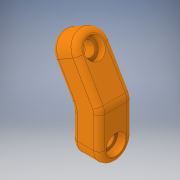
# Autodesk Inventor part: Link2
Saved by Autodesk Inventor 2019 (Build 230136000, 136)
## iProperties
Created: 2022-07-14
Part Number: Link2
Material: Generic
Document SubType Name: Modeling
Designer: zreik
Density: 1 g/cm^3
Appearance: Orange
d46: 10.000 mm
Author: zreik
Autodesk Inventor part; units mm, degrees
ref_plane "YZ Plane" through (0, 0, 0) normal (1, 0, 0) x (0, 1, 0)
ref_plane "XZ Plane" through (0, 0, 0) normal (0, 1, 0) x (-1, 0, 0)
ref_plane "XY Plane" through (0, 0, 0) normal (0, 0, 1) x (1, 0, 0)
sketch "Sketch1" plane through (0, 0, 0) normal (0, 0, 1) x (1, 0, 0)
  line L0 (53.3205, 0) -> (0, 0)
  line L1 (0, 0) -> (60.3287, 34.8308)
  line L2 (43.3205, 0) -> (43.3205, 8.6603)
  line L3 (42.6506, 11.1603) -> (36.8205, 21.2583)
  line L4 (53.3205, 0) -> (53.3205, 11.3397)
  line L5 (52.6506, 13.8397) -> (45.4808, 26.2583)
  arc A0 (43.3205, 8.6603) -> (42.6506, 11.1603) centre (38.3205, 8.6603) ccw
  arc A1 (53.3205, 11.3397) -> (52.6506, 13.8397) centre (48.3205, 11.3397) ccw
  line L6 (45.4808, 26.2583) -> (36.8205, 21.2583)
  line L7 (45.4808, 26.2583) -> (52.6506, 13.8397)
  line L8 (36.8205, 21.2583) -> (42.6506, 11.1603)
  line L9 (43.3205, 0) -> (53.3205, 0)
  line L10 (53.3205, 0) -> (53.3205, 11.3397)
  line L11 (43.3205, 0) -> (53.3205, 0)
  line L12 (53.3205, 0) -> (53.3205, 11.3397)
  line L13 (52.6506, 13.8397) -> (45.4808, 26.2583)
  line L14 (45.4808, 26.2583) -> (36.8205, 21.2583)
  line L15 (36.8205, 21.2583) -> (42.6506, 11.1603)
  line L16 (43.3205, 8.6603) -> (43.3205, 0)
  point P0 (43.3013, 25)
  point P1 (43.3205, 10)
  dimension "d37" = 30
  dimension "d38" = 10
  dimension "d39" = 10
  dimension "d40" = 0
  dimension "d41" = 0
  dimension "d42" = 10
  dimension "d43" = 13
  dimension "d44" = 150
  dimension "d45" = 5
  constraints: 34 end point, 9 collinear, 6 point on line, 4 point on circle, 4 tangent, 2 centre point, 2 parallel, 1 coincident, 1 equal radius, 1 horizontal, 1 vertical
  measures "d37" angle of L1 L0
  measures "d38" distance between parallel lines of L3 L5
  measures "d39" distance between parallel lines of L4 L2
  measures "d40" distance from line of L1 L3.end
  measures "d41" distance from line of L1 L5.end
  measures "d42" distance of L2.start point (43.321, 10)
  measures "d43" distance of point (43.321, 10) L3.end
  measures "d44" angle of L2 L3
  measures "d45" radius of A0
extrude "Extrusion1" add sketch "Sketch1" along normal blind 12 contours L0 L2 A0 L3 L1 L5 A1 L4
ref_plane "Work Plane1" through (52.6506, 13.8397, 0) normal (0.8660254, 0.5, 0) x (-0.5, 0.8660254, 0)
sketch "Sketch2" plane through (52.6506, 13.8397, 0) normal (0.8660254, 0.5, 0) x (-0.5, 0.8660254, 0)
  circle A0 centre (14.3397, 6) radius 6
  line L0 (14.3397, 0) -> (14.3397, 12) projected
  line L1 (0, 12) -> (14.3397, 12) projected
  dimension "d5" = 12
  dimension "d47" = 0
  dimension "d48" = 6
  constraints: 1 centre point
  measures "d5" diameter of A0
  measures "d47" distance from line of L0 A0.centre
  measures "d48" distance from line of L1 A0.centre
extrude "Extrusion2" add sketch "Sketch2" against normal blind 10
ref_plane "Work Plane2" through (53.3205, 11.3397, 0) normal (1, 0, 0) x (0, 1, 0)
sketch "Sketch3" plane through (53.3205, 11.3397, 0) normal (1, 0, 0) x (0, 1, 0)
  circle A0 centre (-11.3397, 6) radius 6
  line L0 (-11.3397, 0) -> (-11.3397, 12) projected
  line L1 (-11.3397, 0) -> (0, 0) projected
  point P0 (43.3013, 10)
  point P1 (9.9186, 12)
  dimension "d10" = 12
  dimension "d49" = 0
  dimension "d50" = 6
  constraints: 1 centre point, 1 other
  measures "d10" diameter of A0
  measures "d49" distance from line of L0 A0.centre
  measures "d50" distance from line of L1 A0.centre
extrude "Extrusion3" add sketch "Sketch3" against normal blind 10
sketch "Sketch4" plane through (43.9904, 8.8397, 0) normal (-0.8660254, -0.5, 0) x (0.5, -0.8660254, 0)
  circle A0 centre (-14.3397, 6) radius 2.5
  circle A1 centre (-14.3397, 6) radius 6 projected
  point P0 (-14.3397, 0)
  point P1 (-14.3397, 12)
  dimension "d15" = 5
  constraints: 1 centre point, 1 concentric
  measures "d15" diameter of A0
extrude "Extrusion4" cut sketch "Sketch4" along normal through all both and the other way through all contours A0
sketch "Sketch5" plane through (43.3205, 11.3397, 0) normal (-1, 0, 0) x (0, 0, 1)
  circle A0 centre (6, -11.3397) radius 2.5
  arc A1 (0, -11.3397) -> (12, -11.3397) centre (6, -11.3397) ccw projected
  dimension "d18" = 5
  constraints: 1 centre point, 1 concentric
  measures "d18" diameter of A0
extrude "Extrusion5" cut sketch "Sketch5" along normal through all both and the other way through all
sketch "Sketch6" plane through (52.6506, 13.8397, 0) normal (0.8660254, 0.5, 0) x (0.5, -0.8660254, 0)
  circle A0 centre (-14.3397, -6) radius 3.6
  circle A1 centre (-14.3397, -6) radius 2.5
  arc A2 (-14.3397, 0) -> (-14.3397, 0) centre (-14.3397, -6) ccw projected
  point P0 (0, -10)
  dimension "d21" = 5
  dimension "d22" = 7.2
  constraints: 2 centre point, 1 coincident, 2 other
  measures "d21" diameter of A1
  measures "d22" diameter of A0
extrude "Extrusion6" cut sketch "Sketch6" against normal blind 3 contours A0
sketch "Sketch7" plane through (43.9904, 8.8397, 0) normal (-0.8660254, -0.5, 0) x (0.5, -0.8660254, 0)
  circle A0 centre (-14.3397, 6) radius 3.6
  circle A1 centre (-14.3397, 6) radius 2.5
  arc A2 (-11.8397, 6) -> (-11.8397, 6) centre (-14.3397, 6) ccw projected
  point P0 (-14.3397, 0)
  dimension "d25" = 5
  dimension "d26" = 7.2
  constraints: 2 centre point, 1 coincident, 1 concentric
  measures "d25" diameter of A1
  measures "d26" diameter of A0
extrude "Extrusion7" cut sketch "Sketch7" along normal mid plane 6
sketch "Sketch8" plane through (43.3205, 11.3397, 0) normal (-1, 0, 0) x (0, 0, 1)
  circle A0 centre (6, -11.3397) radius 3.6
  circle A1 centre (6, -11.3397) radius 2.5
  arc A2 (8.5, -11.3397) -> (8.5, -11.3397) centre (6, -11.3397) ccw projected
  point P0 (0, -11.3397)
  dimension "d29" = 7.2
  dimension "d30" = 5
  constraints: 2 centre point, 1 coincident, 1 concentric
  measures "d29" diameter of A0
  measures "d30" diameter of A1
extrude "Extrusion8" cut sketch "Sketch8" along normal mid plane 6
sketch "Sketch9" plane through (53.3205, 11.3397, 0) normal (1, 0, 0) x (0, 0, -1)
  circle A0 centre (-6, -11.3397) radius 3.6
  circle A1 centre (-6, -11.3397) radius 2.5
  circle A2 centre (-6, -11.3397) radius 2.5 projected
  point P0 (0, -11.3397)
  dimension "d33" = 5
  dimension "d34" = 7.2
  constraints: 2 centre point, 1 coincident, 1 concentric
  measures "d33" diameter of A1
  measures "d34" diameter of A0
extrude "Extrusion9" cut sketch "Sketch9" against normal blind 3
fillet "Fillet1" radius 2 16 edges at (42.4808, 31.4545, 6) (49.0657, 20.049, 0) (53.1501, 12.6338, 0) (53.3205, 5.6699, 0) (53.3205, -6, 6) (53.3205, 5.6699, 12) (53.1501, 12.6338, 12) (49.0657, 20.049, 12) (43.1501, 9.9543, 12) (43.3205, 4.3301, 12) (43.3205, -6, 6) (43.3205, 4.3301, 0) (43.1501, 9.9543, 0) (39.7356, 16.2093, 0) (33.8205, 26.4545, 6) (39.7356, 16.2093, 12)
equation "\"d38\" = d46"
equation "\"d39\" = d46"
equation "\"d3\" = width"
equation "\"d5\" = width"
equation "\"d48\" = 0.5 * width"
equation "\"d8\" = thickness"
equation "\"d10\" = width"
equation "\"d50\" = 0.5 * width"
equation "\"d13\" = thickness"
equation "\"thickness\" = 10"
equation "\"width\" = 12"
equation "\"d46\" = 10"
body "Solid1"
